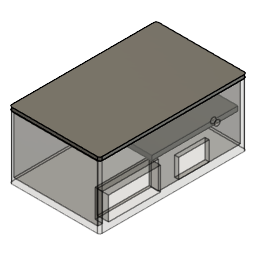
UPS case (Autodesk Fusion 360 design; units mm, degrees)
Autodesk Fusion 360 part; units mm, degrees
note: some values were not read from the file. Chosen so that the rebuilt part matches the saved one: which bodies a step acts on.
sketch "Sketch1" plane through (0, 0, 0) normal (0, 1, 0) x (1, 0, 0)
  line L0 (0, 0) -> (36, 0)
  line L1 (36, 0) -> (36, -38)
  line L2 (36, -38) -> (0, -38)
  line L3 (0, -38) -> (0, 0)
  line L4 (0, 0) -> (0, -6.5)
  line L5 (0, -6.5) -> (7, -6.5)
  line L6 (7, -6.5) -> (7, -15.5)
  line L7 (7, -15.5) -> (0, -15.5)
  line L8 (0, -15.5) -> (0, -6.5)
  dimension "d1" = 36
  dimension "d2" = 38
  dimension "d3" = 6.5
  dimension "d4" = 7
  dimension "d5" = 9
  constraint horizontal L0
  constraint vertical L1
  constraint horizontal L2
  constraint vertical L3
  constraint coincident L0.start L3.end
  constraint perpendicular L0 L4
  constraint horizontal L5
  constraint vertical L6
  constraint horizontal L7
  constraint vertical L8
  measures "d1" distance of L0.start L0.end
  measures "d2" distance of L0.start L2.end
  measures "d3" distance of L0.start L4.end
  measures "d4" distance of L4.end L5.end
  measures "d5" distance of L4.end L7.end
extrude "Extrude1" add sketch "Sketch1" along normal blind 3 contours L3 L5 L6 L7 L8 makes body 1
extrude "Extrude2" add sketch "Sketch1" against normal blind 2 separate body contours L0 L1 L2 L3 L4 L5 L6 L7 makes body 2
extrude "Extrude3" add sketch "Sketch1" against normal blind 2 contours L3 L5 L6 L7 L8 bodies 1 2
fillet "Fillet1" radius 1 2 edges at (3.5, 3, 6.5) (3.5, 3, 15.5) on bodies 1
sketch "Sketch2" plane through (0, 0, 0) normal (0, 1, 0) x (1, 0, 0)
  line L0 (40, 0) -> (63, 0)
  line L1 (63, 0) -> (63, -60)
  line L2 (63, -60) -> (40, -60)
  line L3 (40, -60) -> (40, 0)
  dimension "d14" = 23
  dimension "d15" = 60
  constraint horizontal L0
  constraint vertical L1
  constraint horizontal L2
  constraint vertical L3
  measures "d14" distance of L0.start L0.end
  measures "d15" distance of L0.start L2.end
extrude "Extrude4" add sketch "Sketch2" along normal blind 10 separate body makes body 3
move_body "Move1" bodies 3 to x (1, 0, 0) y (0, 1, 0) z (0, 0, 1) at (0, -12.6, 0)
move_body "Move2" bodies 3 to x (1, 0, 0) y (0, 1, 0) z (0, 0, 1) at (-39, 0, 0)
sketch "Sketch3" plane through (0, 0, 0) normal (0, 1, 0) x (1, 0, 0)
  line L0 (0, 0) -> (37, 0)
  line L1 (37, 0) -> (37, -61)
  line L2 (37, -61) -> (0, -61)
  line L3 (0, -61) -> (0, 0)
  line L4 (-1, 2) -> (39, 2)
  line L5 (39, 2) -> (39, -63)
  line L6 (39, -63) -> (-1, -63)
  line L7 (-1, -63) -> (-1, 2)
  constraint horizontal L0
  constraint vertical L1
  constraint horizontal L2
  constraint vertical L3
  constraint coincident L0.start L3.end
  constraint horizontal L4
  constraint vertical L5
  constraint horizontal L6
  constraint vertical L7
extrude "Extrude5" add sketch "Sketch3" against normal blind 15 separate body makes body 4
extrude "Extrude6" add 1 faces at (38.3333, 0, 40.6667) along direction (0, 1, 0) blind 7 on bodies 4 bodies 4
sketch "Sketch4" plane through (-1, 0, 0) normal (-1, 0, 0) x (0, 0, 1)
  line L0 (-2, 7) -> (-2, -15)
  line L1 (-2, -15) -> (63, -15)
  line L2 (63, -15) -> (63, 7)
  line L3 (63, 7) -> (-2, 7)
  line L4 (6.5, 3) -> (15.5, 3)
  line L5 (15.5, 3) -> (15.5, 0)
  line L6 (15.5, 0) -> (6.5, 0)
  line L7 (6.5, 0) -> (6.5, 3)
  constraint horizontal L4
  constraint vertical L5
  constraint horizontal L6
  constraint vertical L7
extrude "Extrude7" cut sketch "Sketch4" against normal blind 1 contours L4 L5 L6 L7 bodies 4
fillet "Fillet2" radius 0.8 4 edges at (-0.5, 3, 6.5) (-0.5, 3, 15.5) (-0.5, 0, 15.5) (-0.5, 0, 6.5) on bodies 4
sketch "Sketch5" plane through (39, 0, 0) normal (1, 0, 0) x (0, 0, -1)
  line L0 (-63, 7) -> (-63, -15)
  line L1 (-63, -15) -> (2, -15)
  line L2 (2, -15) -> (2, 7)
  line L3 (2, 7) -> (-63, 7)
  line L4 (-59.1322, -3.9623) -> (-36.1322, -3.9623)
  line L5 (-36.1322, -3.9623) -> (-36.1322, -13.9623)
  line L6 (-36.1322, -13.9623) -> (-59.1322, -13.9623)
  line L7 (-59.1322, -13.9623) -> (-59.1322, -3.9623)
  line L8 (-60, -3) -> (-35.2458, -3)
  line L9 (-35.2458, -3) -> (-35.2458, -15)
  line L10 (-35.2458, -15) -> (-60, -15)
  line L11 (-60, -15) -> (-60, -3)
  dimension "d26" = 23
  dimension "d27" = 10
  constraint horizontal L4
  constraint vertical L5
  constraint horizontal L6
  constraint vertical L7
  constraint horizontal L8
  constraint vertical L9
  constraint horizontal L10
  constraint vertical L11
  constraint coincident L1 L9.end
  measures "d26" distance of L4.start L4.end
  measures "d27" distance of L4.start L6.end
extrude "Extrude8" add sketch "Sketch5" against normal blind 6 contours L1 L8 L9 L10 L11 bodies 4
sketch "Sketch6" plane through (0, -15, 0) normal (0, -1, 0) x (1, 0, 0)
  line L0 (39, -2) -> (39, 63)
  line L1 (39, 63) -> (-1, 63)
  line L2 (-1, 63) -> (-1, -2)
  line L3 (-1, -2) -> (39, -2)
  line L4 (37, 35.2458) -> (37, 0)
  line L5 (37, 0) -> (0, 0)
  line L6 (0, 0) -> (0, 61)
  line L7 (0, 61) -> (37, 61)
  line L8 (37, 61) -> (37, 60)
  line L9 (37, 60) -> (33, 60)
  line L10 (33, 60) -> (33, 35.2458)
  line L11 (33, 35.2458) -> (37, 35.2458)
  line L12 (39, 63) -> (-1, 63)
  line L13 (-1, 63) -> (-1, -2)
  line L14 (-1, -2) -> (39, -2)
  line L15 (39, -2) -> (39, 63)
  constraint horizontal L12
  constraint vertical L13
  constraint horizontal L14
  constraint vertical L15
  constraint coincident L2.end L3.start
  constraint coincident L0.end L1.start
extrude "Extrude9" add sketch "Sketch6" along normal blind 2 contours L0 L1 L2 L3 L12 L13 L14 L15 | L4 L5 L6 L7 L8 L9 L10 L11 bodies 4
extrude "Extrude10" cut sketch "Sketch5" against normal blind 2 contours L4 L5 L6 L7 bodies 4
sketch "Sketch7" plane through (39, 0, 0) normal (1, 0, 0) x (0, 0, -1)
  line L0 (-28.0861, -4.7174) -> (-15.0861, -4.7174)
  line L1 (-15.0861, -4.7174) -> (-15.0861, -12.7174)
  line L2 (-15.0861, -12.7174) -> (-28.0861, -12.7174)
  line L3 (-28.0861, -12.7174) -> (-28.0861, -4.7174)
  circle A0 centre (-11, 0) radius 1.75
  dimension "d34" = 13
  dimension "d35" = 8
  dimension "d36" = 3.5
  constraint horizontal L0
  constraint vertical L1
  constraint horizontal L2
  constraint vertical L3
  measures "d34" distance of L0.start L0.end
  measures "d35" distance of L0.start L2.end
  measures "d36" diameter of A0
extrude "Extrude11" cut sketch "Sketch7" against normal blind 2 bodies 4
extrude "Extrude12" cut sketch "Sketch5" against normal blind 1 contours L0 L1 L2 L3 L8 L9 L11 bodies 4
extrude "Extrude13" cut 1 faces at (39, -16.3333, 32.0819) along direction (-1, 0, 0) blind 1 on bodies 4 bodies 4
move_face "OffsetFaces1" offset 0.5 1 faces at (37.6667, -0.1742, 9.2587) on bodies 4
sketch "Sketch8" plane through (0, 7, 0) normal (0, 1, 0) x (-1, 0, 0)
  line L0 (-38, 63) -> (-38, -2)
  line L1 (-38, -2) -> (1, -2)
  line L2 (1, -2) -> (1, 63)
  line L3 (1, 63) -> (-38, 63)
  line L4 (-37, 61) -> (0, 61)
  line L5 (0, 61) -> (0, 0)
  line L6 (0, 0) -> (-37, 0)
  line L7 (-37, 0) -> (-37, 61)
  line L8 (-38, 63) -> (1, 63)
  line L9 (1, 63) -> (1, -2)
  line L10 (1, -2) -> (-38, -2)
  line L11 (-38, -2) -> (-38, 63)
  line L12 (-37, 61) -> (0, 61)
  line L13 (0, 61) -> (0, 0)
  line L14 (0, 0) -> (-37, 0)
  line L15 (-37, 0) -> (-37, 61)
  line L16 (-35.6939, 59.5295) -> (-1.3777, 59.5295)
  line L17 (-1.3777, 59.5295) -> (-1.3777, 1.4686)
  line L18 (-1.3777, 1.4686) -> (-35.6939, 1.4686)
  line L19 (-35.6939, 1.4686) -> (-35.6939, 59.5295)
  constraint horizontal L8
  constraint vertical L9
  constraint horizontal L10
  constraint vertical L11
  constraint coincident L1.end L2.start
  constraint coincident L0.start L3.end
  constraint horizontal L12
  constraint vertical L13
  constraint horizontal L14
  constraint vertical L15
  constraint coincident L5.end L6.start
  constraint coincident L4.start L7.end
  constraint horizontal L16
  constraint vertical L17
  constraint horizontal L18
  constraint vertical L19
extrude "Extrude14" add sketch "Sketch8" along normal blind 1.5 separate body contours L0 L1 L2 L3 L8 L9 L10 L11 | L4 L5 L6 L7 L12 L13 L14 L15 | L16 L17 L18 L19 makes body 5
extrude "Extrude15" add sketch "Sketch8" against normal blind 2 contours L4 L5 L6 L7 L12 L13 L14 L15 bodies 5
chamfer "Chamfer1" distance 0.6 angle 45 4 edges at (18.5, 5, 0) (0, 5, 30.5) (37, 5, 30.5) (18.5, 5, 61) on bodies 5
fillet "Fillet3" radius 1 8 edges at (38, -5, 63) (38, -5, -2) (-1, -5, -2) (-1, -5, 63) (38, 7.75, 63) (38, 7.75, -2) (-1, 7.75, -2) (-1, 7.75, 63) on bodies 4 5
move_face "OffsetFaces2" offset -0.3 1 faces at (34.6667, -3.9623, 51.4655) on bodies 4
extrude "Extrude16" add 1 faces at (34.3333, -3, 43.4972) along direction (0, 1, 0) blind 0.3 on bodies 4 bodies 4
move_face "OffsetFaces3" offset -0.5 2 faces at (37.3333, -12.7174, 19.4194) (37.6667, -7.3841, 15.0861) on bodies 4
extrude "Extrude17" cut 1 faces at (12.3333, -7.6667, 61) along direction (0, 0, 1) blind 1 on bodies 4 bodies 4
extrude "Extrude18" cut 1 faces at (24.6667, -7.6667, 0) along direction (0, 0, -1) blind 1 on bodies 4 bodies 4
sketch "Sketch9" plane through (0, 7, 0) normal (0, 1, 0) x (-1, 0, 0)
  arc A0 (1, 62) -> (0, 63) centre (0, 62) ccw
  line L0 (0, 63) -> (-37, 63)
  arc A1 (-37, 63) -> (-38, 62) centre (-37, 62) ccw
  line L1 (-38, 62) -> (-38, -1)
  arc A2 (-38, -1) -> (-37, -2) centre (-37, -1) ccw
  line L2 (-37, -2) -> (0, -2)
  arc A3 (0, -2) -> (1, -1) centre (0, -1) ccw
  line L3 (1, -1) -> (1, 62)
  line L4 (0, 62) -> (0, -1)
  line L5 (0, -1) -> (-37, -1)
  line L6 (-37, -1) -> (-37, 62)
  line L7 (-37, 62) -> (0, 62)
  line L8 (0, -2) -> (2, -2)
  line L9 (2, -2) -> (2, 63)
  line L10 (2, 63) -> (0, 63)
  line L11 (0, 63) -> (0, -2)
  constraint horizontal L8
  constraint vertical L9
  constraint horizontal L10
  constraint vertical L11
  constraint coincident L2.end A3.start
extrude "Extrude19" add sketch "Sketch9" against normal blind 24 contours A0 A3 L3 L8 L9 L10 bodies 4
extrude "Extrude20" cut 1 faces at (0, -2.4417, 46.4967) along direction (-1, 0, 0) blind 1 on bodies 4 bodies 4
fillet "Fillet4" radius 1 2 edges at (-2, -5, -2) (-2, -5, 63) on bodies 4
extrude "Extrude21" add sketch "Sketch9" along normal blind 1.5 contours A0 A3 L3 L8 L9 L10 bodies 5
extrude "Extrude22" add sketch "Sketch8" against normal blind 2 contours L4 L5 L6 L7 L12 L13 L14 L15 bodies 5
extrude "Extrude23" add 1 faces at (0, 6.3333, 40.6667) along direction (-1, 0, 0) blind 1 on bodies 5 bodies 5
extrude "Extrude24" cut 1 faces at (1.3777, 5.6667, 40.1759) along direction (-1, 0, 0) blind 1 on bodies 5 bodies 5
fillet "Fillet5" radius 1 2 edges at (-2, 7.75, -2) (-2, 7.75, 63) on bodies 5
chamfer "Chamfer2" distance 0.8 angle 45 4 edges at (-1, 5, 30.5) (18, 5, 61) (18, 5, 0) (37, 5, 30.5) on bodies 5
extrude "Extrude25" cut sketch "Sketch4" along normal blind 4 contours L4 L5 L6 L7 bodies 4
fillet "Fillet6" radius 0.8 4 edges at (-1.5, 3, 6.5) (-1.5, 0, 6.5) (-1.5, 0, 15.5) (-1.5, 3, 15.5) on bodies 4
extrude "Extrude26" cut 1 faces at (12.1259, 5, 59.9765) along direction (0, 1, 0) blind 2 on bodies 5 bodies 5
extrude "Extrude27" cut 1 faces at (11.9333, 5.6667, 0.8) along direction (0, 0, -1) blind 6 on bodies 5 bodies 5
extrude "Extrude28" cut 1 faces at (-1, 6.2, 20.3333) along direction (1, 0, 0) blind 60 on bodies 5 bodies 5 makes body 6 at (-0.7333, 5.8, 40.4)
extrude "Extrude29" cut 1 faces at (-0.7333, 5.8, 40.4) along direction (0, -1, 0) blind 4 on bodies 6 bodies 6
sketch "Sketch10" plane through (0, 7, 0) normal (0, -1, 0) x (1, 0, 0)
  line L0 (38, -1) -> (38, 62)
  arc A0 (38, 62) -> (37, 63) centre (37, 62) ccw
  line L1 (37, 63) -> (-1, 63)
  arc A1 (-1, 63) -> (-2, 62) centre (-1, 62) ccw
  line L2 (-2, 62) -> (-2, -1)
  arc A2 (-2, -1) -> (-1, -2) centre (-1, -1) ccw
  line L3 (-1, -2) -> (37, -2)
  arc A3 (37, -2) -> (38, -1) centre (37, -1) ccw
  line L4 (37, -1) -> (-1, -1)
  line L5 (-1, -1) -> (-1, 62)
  line L6 (-1, 62) -> (37, 62)
  line L7 (37, 62) -> (37, -1)
  line L8 (35.5, 0.5) -> (0.5, 0.5)
  line L9 (0.5, 0.5) -> (0.5, 60.5)
  line L10 (0.5, 60.5) -> (35.5, 60.5)
  line L11 (35.5, 60.5) -> (35.5, 0.5)
  constraint horizontal L4
  constraint vertical L5
  constraint horizontal L6
  constraint vertical L7
  constraint coincident A1.centre L5.end
  constraint coincident A3.centre L4.start
  constraint horizontal L8
  constraint vertical L9
  constraint horizontal L10
  constraint vertical L11
delete_body "RemoveBody1" bodies 6
extrude "Extrude30" add sketch "Sketch10" along normal blind 2 contours L4 L5 L6 L7 bodies 5
extrude "Extrude31" add 1 faces at (35.5, 6.3333, 40.5) along direction (-1, 0, 0) blind 0.8 on bodies 5 bodies 5
extrude "Extrude32" cut 1 faces at (37, 6.3333, 41) along direction (-1, 0, 0) blind 0.8 on bodies 5 bodies 5
extrude "Extrude33" add 1 faces at (37, -2.7895, 2.6018) along direction (-1, 0, 0) blind 0.8 on bodies 4 bodies 4
chamfer "Chamfer3" distance 0.8 angle 45 4 edges at (36.2, 5, 30.5) (17.6, 5, -1) (-1, 5, 30.5) (17.6, 5, 62) on bodies 5
extrude "Extrude34" add 1 faces at (37.4, 7, 20) along direction (0, 1, 0) blind 4 separate body on bodies 4 makes body 7
extrude "Extrude35" add 1 faces at (37.4, 7, 20) along direction (0, -1, 0) blind 1 on bodies 7 bodies 4 7
move_body "Move3" bodies 5 to x (1, 0, 0) y (0, 1, 0) z (0, 0, 1) at (0, 4, 0)
hidden bodies 3
named bodies: "Board", "Battery", "Case", "Lid", "Lid (1)"
